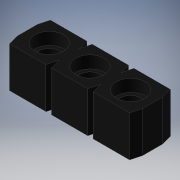
# Autodesk Inventor part: TS-103-G-A_socket
Saved by Autodesk Inventor 2019 (Build 230136000, 136)
## iProperties
Created: 2024-02-02
Part Number: TS-103-G-A_socket
Material: Generic
Catalog Web Link: www.cadenas.de
Description: TS Series Socket-TS Series - (2,54 mm) .100'' Precision Machined Terminal Strips
Vendor: SAMTEC
Document SubType Name: Modeling
Designer: psAdmin
Manufacturer: SAMTEC
Mass: 0.0358414 g
Surface Area: 1.26171 cm^2
Volume: 0.0358414 cm^3
Density: 1 g/cm^3
Appearance: PSOLRGB-127-127-127
Category: PARTsolutions
Company: SAMTEC
Title: TS-103-G-A_socket
Author: Cadenas PARTsolutions
Comments: TS Series - (2,54 mm) .100'' Precision Machined Terminal Strips
PSOL_IDENT_0: {$CADENAS_DATA/23d-libs/samtec/modelling/ts/parts/ts_socket.prj},200 {VTYP=3D},{NB=TS-103-G-A_socket
PSOL_IDENT_1: },{LINA=TS-103-G-A_socket},{NN=TS Series Socket},{DATE=03.10.2016 09:07:49},{GEOMDATE=03.10.2016 09:
PSOL_IDENT_2: 01:00},{VERSION=},{LINEID=10},{WBVAR=ROW,POS,PLOPT,LS},{WBNUMERIC=}  {NB=TS-103-G-A_socket},{LINA=TS
PSOL_IDENT_3: -103-G-A_socket},{KT=DUMMY},{PN=TS-103-G-A},{SERIES=TS},{ROWALG=   'TS' , '-TS = Single Row'  , 'TD'
PSOL_IDENT_4: , '-TD = Double Row'  },{ROW=TS},{POS=03},{POSN=3},{POSALG=  '01','-01','02','-02','03','-03','04','
PSOL_IDENT_5: -04','05','-05','06','-06','07','-07','08','-08','09','-09','10','-10','11','-11','12','-12','13','-
PSOL_IDENT_6: 13','14','-14','15','-15','16','-16','17','-17','18','-18','19','-19','20','-20','21','-21','22','-2
PSOL_IDENT_7: 2','23','-23','24','-24','25','-25','26','-26','27','-27','28','-28','29','-29','30','-30','31','-31'
PSOL_IDENT_8: ,'32','-32' },{POSPN=03},{PLOPT=G},{PLOPTALG=  'G' , '-G = 20micro\" Selective Gold.'   },{LS=A},{LS
PSOL_IDENT_9: ALG= 'AA','-AA','A','-A','A-1','-A-1','A-2','-A-2','B','-B','B-2','-B-2','C','-C','C-1','-C-1','C-2'
PSOL_IDENT_10: ,'-C-2','D-1-1','-D-1-1','D-1-2','-D-1-2','E','-E','G-1','-G-1','J','-J','K','-K','L-1','-L-1','L-2'
PSOL_IDENT_11: ,'-L-2','L-3','-L-3','N','-N','Q-3','-Q-3' },{FIG=2},{A=0.100},{B=0.1},{C=0.143},{D=0.018},{D2=0.018
PSOL_IDENT_12: },{E=0.156},{F=0.166},{G=0.008},{H=0.070},{I=0.052},{J=0.052},{PL=0.477},{SQ=0.000},{W=0.30800},{X=0
PSOL_IDENT_13: },{EVEN=0.000}
NB: TS-103-G-A_socket
NN: TS Series Socket
NT: TS Series - (2,54 mm) .100'' Precision Machined Terminal Strips
NBSYN: $PN._socket
LINA: TS-103-G-A_socket
CATALOG: Samtec
PN: TS-103-G-A
SERIES: TS
ROW: -TS = Single Row
POS: -03
PLOPT: -G = 20micro" Selective Gold.
LS: -A
FIG: 2
A: 0.1
B: 0.1
C: 0.143
D: 0.018
D2: 0.018
E: 0.156
F: 0.166
G: 0.008
H: 0.07
I: 0.052
J: 0.052
PL: 0.477
SQ: 0
W: 0.308
SUPPLIER: SAMTEC
ARTICLENO: TS-103-G-A_socket
BOMINFO: TS-103-G-A_socket
CREATOR: CADENAS GmbH
Autodesk Inventor part; units mm, degrees
sketch "Sketch_17" plane through (0, 0, 0) normal (0, 1, 0) x (-1, 0, 0)
  line L0 (-0.254, -0.635) -> (-0.254, 0.635)
  line L1 (-0.254, 0.635) -> (-7.5692, 0.635)
  line L2 (-7.5692, 0.635) -> (-7.5692, -0.635)
  line L3 (-7.5692, -0.635) -> (-0.254, -0.635)
  constraints: 8 end point
extrude "Extrusion1" add sketch "Sketch_17" along normal blind 2.54
sketch "Sketch_3" plane through (0, 0, 0) normal (0, 1, 0) x (-1, 0, 0)
  line L0 (0, 0.635) -> (-0.1701, 1.27)
  line L1 (-0.1701, 1.27) -> (-2.4376, 1.27)
  line L2 (-2.4376, 1.27) -> (-2.6077, 0.635)
  line L3 (-2.6077, 0.635) -> (-2.6077, -0.635)
  line L4 (-2.6077, -0.635) -> (-2.4376, -1.27)
  line L5 (-2.4376, -1.27) -> (-0.1701, -1.27)
  line L6 (-0.1701, -1.27) -> (0, -0.635)
  line L7 (0, -0.635) -> (0, 0.635)
  constraints: 16 end point
extrude "Extrusion2" add sketch "Sketch_3" along normal blind 2.54
pattern_linear "Rectangular Pattern1" count 3 spacing 2.6077 along (1, 0, 0) of "Extrusion2"
sketch "Sketch3" plane through (0, 0, 0) normal (0, -1, 0) x (1, 0, 0)
  point P0 (1.3716, 0)
hole "Hole1" at (1.3716, 0, 0) direction (0, 1, 0) diameter 1.3208 depth 2.54
pattern_linear "Rectangular Pattern2" count 3 spacing 2.54 along (1, 0, 0) of "Hole1"
sketch "Sketch_7" plane through (0, 2.54, 0) normal (0, 1, 0) x (1, 0, 0)
  circle A0 centre (1.3716, 0) radius 0.889
  constraints: 1 centre point
extrude "Extrusion3" cut sketch "Sketch_7" against normal blind 0.762
pattern_linear "Rectangular Pattern3" count 3 spacing 2.54 along (1, 0, 0) of "Extrusion3"
ref_plane "socket_XY" through (3.9116, 0, 0) normal (0, 1, 0) x (1, 0, 0)
ref_plane "socket_YZ" through (3.9116, 0, 0) normal (1, 0, 0) x (0, 0, -1)
ref_plane "socket_ZX" through (3.9116, 0, 0) normal (0, 0, -1) x (0, 1, 0)
ref_plane "to_pin_1_XY" through (1.3716, 2.7432, 0) normal (0, 1, 0) x (1, 0, 0)
ref_plane "to_pin_1_YZ" through (1.3716, 2.7432, 0) normal (1, 0, 0) x (0, 0, -1)
ref_plane "to_pin_1_ZX" through (1.3716, 2.7432, 0) normal (0, 0, -1) x (0, 1, 0)
ref_plane "to_pin_2_XY" through (3.9116, 2.7432, 0) normal (0, 1, 0) x (1, 0, 0)
ref_plane "to_pin_2_YZ" through (3.9116, 2.7432, 0) normal (1, 0, 0) x (0, 0, -1)
ref_plane "to_pin_2_ZX" through (3.9116, 2.7432, 0) normal (0, 0, -1) x (0, 1, 0)
ref_plane "to_pin_3_XY" through (6.4516, 2.7432, 0) normal (0, 1, 0) x (1, 0, 0)
ref_plane "to_pin_3_YZ" through (6.4516, 2.7432, 0) normal (1, 0, 0) x (0, 0, -1)
ref_plane "to_pin_3_ZX" through (6.4516, 2.7432, 0) normal (0, 0, -1) x (0, 1, 0)
ref_plane "to_pin2_1_XY" through (1.3716, 2.7432, 0) normal (0, 1, 0) x (1, 0, 0)
ref_plane "to_pin2_1_YZ" through (1.3716, 2.7432, 0) normal (1, 0, 0) x (0, 0, -1)
ref_plane "to_pin2_1_ZX" through (1.3716, 2.7432, 0) normal (0, 0, -1) x (0, 1, 0)
ref_plane "to_pin2_2_XY" through (3.9116, 2.7432, 0) normal (0, 1, 0) x (1, 0, 0)
ref_plane "to_pin2_2_YZ" through (3.9116, 2.7432, 0) normal (1, 0, 0) x (0, 0, -1)
ref_plane "to_pin2_2_ZX" through (3.9116, 2.7432, 0) normal (0, 0, -1) x (0, 1, 0)
ref_plane "to_pin2_3_XY" through (6.4516, 2.7432, 0) normal (0, 1, 0) x (1, 0, 0)
ref_plane "to_pin2_3_YZ" through (6.4516, 2.7432, 0) normal (1, 0, 0) x (0, 0, -1)
ref_plane "to_pin2_3_ZX" through (6.4516, 2.7432, 0) normal (0, 0, -1) x (0, 1, 0)
body "Solid1"
